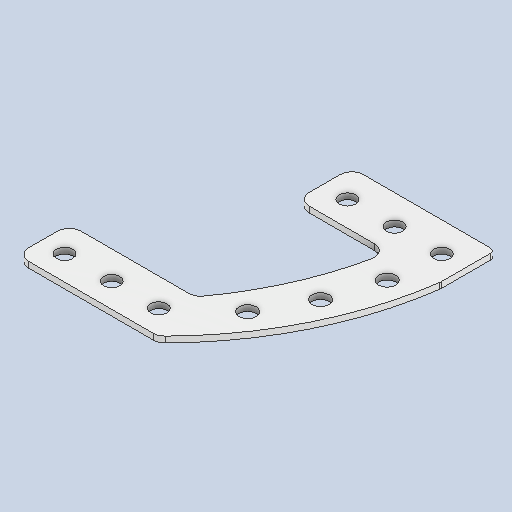
# Autodesk Inventor part: Drive_Bumpers
Saved by Autodesk Inventor 2025.2 (Build 292293000, 293)
## iProperties
Created: 2024-12-08
Part Number: Drive_Bumpers
Material: Acetal Resin, White
Document SubType Name: Modeling
Designer: Aditya Koduri
Density: 1.425 g/cm^3
Appearance: Smooth - White
Mass: 3.58172 g
Surface Area: 37.9184 cm^2
Volume: 2.51349 cm^3
Author: Aditya Koduri
Autodesk Inventor part; units mm, degrees
ref_plane "YZ Plane" through (0, 0, 0) normal (1, 0, 0) x (0, 1, 0)
ref_plane "XZ Plane" through (0, 0, 0) normal (0, 1, 0) x (-1, 0, 0)
ref_plane "XY Plane" through (0, 0, 0) normal (0, 0, 1) x (1, 0, 0)
sketch "Sketch1" plane through (0, 0, 0) normal (0, 1, 0) x (-1, 0, 0)
  circle A0 centre (-13.1748, 27.6836) radius 2.1844
  circle A1 centre (-0.4748, 27.6836) radius 2.1844
  circle A2 centre (12.2252, 27.6836) radius 2.1844
  circle A3 centre (-38.5746, -23.1179) radius 2.1844
  circle A4 centre (-25.8746, -23.1179) radius 2.1844
  circle A5 centre (-13.1746, -23.1178) radius 2.1844
  line L0 (-18.5197, 34.2524) -> (-18.2507, 34.2524)
  line L1 (-18.5197, 34.2524) -> (15.3028, 34.2524)
  line L2 (18.4778, 31.0774) -> (18.4778, 23.3345)
  line L3 (15.3028, 20.1595) -> (-13.7382, 20.1595)
  arc A6 (-16.3086, 18.8482) -> (-30.2816, -12.5795) centre (50.793, -29.8056) ccw
  line L4 (-27.1759, -16.4144) -> (-9.5634, -16.4144)
  line L5 (-6.3884, -19.5894) -> (-6.3884, -27.8836)
  line L6 (-9.5634, -31.0586) -> (-43.7283, -31.0586)
  line L7 (-44.9983, -29.7886) -> (-44.9983, -16.6308)
  arc A7 (-20.5068, 33.3114) -> (-44.9684, -16.196) centre (41.5705, -28.1579) ccw
  arc A8 (-18.2507, 34.2524) -> (-20.5068, 33.3114) centre (-18.2507, 31.0774) ccw
  arc A9 (18.4778, 31.0774) -> (15.3028, 34.2524) centre (15.3028, 31.0774) ccw
  arc A10 (15.3028, 20.1595) -> (18.4778, 23.3345) centre (15.3028, 23.3345) ccw
  arc A11 (-13.7382, 20.1595) -> (-16.3086, 18.8482) centre (-13.7382, 16.9845) ccw
  arc A12 (-30.2816, -12.5795) -> (-27.1759, -16.4144) centre (-27.1759, -13.2394) ccw
  arc A13 (-6.3884, -19.5894) -> (-9.5634, -16.4144) centre (-9.5634, -19.5894) ccw
  arc A14 (-9.5634, -31.0586) -> (-6.3884, -27.8836) centre (-9.5634, -27.8836) ccw
  arc A15 (-44.9684, -16.196) -> (-44.9983, -16.6308) centre (-41.8233, -16.6308) ccw
  arc A16 (-44.9983, -29.7886) -> (-43.7283, -31.0586) centre (-43.7283, -29.7886) ccw
  circle A17 centre (-25.9031, 16.5011) radius 2.3114
  circle A18 centre (-32.9166, 3.8671) radius 2.3114
  circle A19 centre (-37.377, -9.6316) radius 2.3114
  point P0 (0, 0)
  point P1 (-19.5607, 34.2524)
  point P2 (-15.338, 20.1595)
  point P3 (-30.5749, -14.023)
  point P4 (-25.9031, -16.4144)
  point P5 (-44.9983, -16.4144)
  dimension "d0" = 3.175
  dimension "d1" = 3.175
  dimension "d2" = 1.27
  dimension "d3" = 4.6228
  dimension "d4" = 4.6228
  dimension "d5" = 4.6228
  constraints: 26 point on circle, 20 centre point, 18 tangent, 16 end point, 6 equal radius, 5 perpendicular, 5 point on line, 3 horizontal
  measures "d0" radius of A8
  measures "d1" radius of A15
  measures "d2" radius of A16
  measures "d3" diameter of A17
  measures "d4" diameter of A18
  measures "d5" diameter of A19
extrude "Extrusion1" add sketch "Sketch1" along normal blind 1.5875
body "Solid1"
